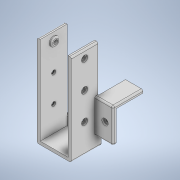
# Autodesk Inventor part: cornerMountTL_PBF
Saved by Autodesk Inventor 2020 (Build 240168000, 168)
## iProperties
Created: 2020-02-06
Part Number: cornerMountTL_PBF
Material: Generic
Document SubType Name: Modeling
Designer: PAB
Density: 1 g/cm^3
Appearance: Default
Author: PAB
Autodesk Inventor part; units mm, degrees
ref_plane "YZ Plane" through (0, 0, 0) normal (1, 0, 0) x (0, 1, 0)
ref_plane "XZ Plane" through (0, 0, 0) normal (0, 1, 0) x (-1, 0, 0)
ref_plane "XY Plane" through (0, 0, 0) normal (0, 0, 1) x (1, 0, 0)
sketch "Sketch1" plane through (0, 0, 0) normal (0, 1, 0) x (-1, 0, 0)
  line L0 (16.2, 12.7) -> (-16.2, 12.7)
  line L1 (-16.2, 12.7) -> (-16.2, -12.7)
  line L2 (-16.2, -12.7) -> (16.2, -12.7)
  line L3 (16.2, -12.7) -> (16.2, 12.7)
  point P0 (0, 0)
  dimension "d0" = 32.4
  dimension "d1" = 25.4
  constraints: 8 end point, 2 parallel, 1 horizontal, 1 perpendicular
  measures "d0" distance of L2.end L1.end
  measures "d1" distance of L1.end L0.end
extrude "Extrusion1" add sketch "Sketch1" along normal blind 3
sketch "Sketch2" plane through (0, 3, 0) normal (0, 1, 0) x (1, 0, 0)
  line L0 (-16.2, 12.7) -> (-16.2, -12.7) projected
  line L1 (16.2, 12.7) -> (-16.2, 12.7) projected
  line L2 (-16.2, -12.7) -> (-13.2, -12.7)
  line L3 (-13.2, -12.7) -> (-13.2, 12.7)
  line L4 (-13.2, 12.7) -> (-16.2, 12.7)
  line L5 (-16.2, 12.7) -> (-16.2, -12.7)
  line L6 (-16.2, -12.7) -> (16.2, -12.7) projected
  line L7 (16.2, 12.7) -> (13.2, 12.7)
  line L8 (13.2, 12.7) -> (13.2, -12.7)
  line L9 (13.2, -12.7) -> (16.2, -12.7)
  line L10 (16.2, -12.7) -> (16.2, 12.7)
  point P0 (0, 0)
  dimension "d4" = 3
  dimension "d5" = 3
  constraints: 16 end point, 4 parallel, 2 horizontal, 2 perpendicular, 2 point on line
  measures "d4" distance of L4.end L3.end
  measures "d5" distance of L9.end L8.end
extrude "Extrusion2" add sketch "Sketch2" along normal blind 83.75 contours L1 L3 L2 L0 | L1 L10 L6 L8
sketch "Sketch3" plane through (16.2, 0, 12.7) normal (1, 0, 0) x (0, 0, -1)
  circle A0 centre (12.7, 79.25) radius 2
  point P0 (12.7, 0)
  dimension "d8" = 4
  constraints: 1 centre point
  measures "d8" diameter of A0
extrude "Extrusion3" cut sketch "Sketch3" against normal blind 3
sketch "Sketch4" plane through (16.2, 0, 12.7) normal (1, 0, 0) x (0, 0, -1)
  circle A0 centre (12.7, 79.25) radius 2 projected
  circle A1 centre (12.7, 79.25) radius 3
  point P0 (12.7, 0)
  dimension "d11" = 6
  constraints: 1 centre point, 1 coincident
  measures "d11" diameter of A1
extrude "Extrusion4" cut sketch "Sketch4" against normal blind 1.5 contours A0 | A1
sketch "Sketch5" plane through (13.2, 3, -12.7) normal (-1, 0, 0) x (0, 0, 1)
  circle A0 centre (12.7, 76.25) radius 2 projected
  circle A1 centre (12.7, 76.25) radius 4.25
  point P0 (12.7, -3)
  dimension "d14" = 8.5
  constraints: 1 centre point, 1 coincident
  measures "d14" diameter of A1
extrude "Extrusion5" add sketch "Sketch5" along normal blind 2
fillet "Fillet1" radius 1.2 1 edges at (11.2, 79.25, -4.25)
pattern_linear "Rectangular Pattern1" count 3 spacing -26 along (0, 1, 0) of "Extrusion3", "Extrusion4"
mirror "Mirror2" about plane through (0, 0, 0) normal (1, 0, 0) of "Extrusion3", "Extrusion4", "Extrusion5", "Fillet1", "Rectangular Pattern1"
sketch "Sketch6" plane through (16.2, 0, 12.7) normal (1, 0, 0) x (0, 0, -1)
  line L0 (25.4, 0) -> (25.4, 86.75) projected
  line L1 (25.4, 43.45) -> (22.4, 43.45)
  line L2 (22.4, 43.45) -> (22.4, 11.05)
  line L3 (22.4, 11.05) -> (25.4, 11.05)
  line L4 (25.4, 11.05) -> (25.4, 43.45)
  point P0 (12.7, 0)
  dimension "d21" = 3
  dimension "d22" = 32.4
  constraints: 8 end point, 2 parallel, 1 horizontal, 1 perpendicular, 1 point on line
  measures "d21" distance of L3.end L2.end
  measures "d22" distance of L2.end L1.end
extrude "Extrusion6" add sketch "Sketch6" along normal blind 17.3
sketch "Sketch7" plane through (16.2, 11.05, -9.7) normal (0, 0, 1) x (1, 0, 0)
  circle A0 centre (9.8, 16.2) radius 2
  point P0 (-16.2, -11.05)
  dimension "d25" = 4
  constraints: 1 centre point
  measures "d25" diameter of A0
extrude "Extrusion7" cut sketch "Sketch7" against normal blind 3
sketch "Sketch8" plane through (16.2, 11.05, -9.7) normal (0, 0, 1) x (1, 0, 0)
  circle A0 centre (9.8, 16.2) radius 2 projected
  circle A1 centre (9.8, 16.2) radius 3
  point P0 (-16.2, -11.05)
  dimension "d28" = 6
  constraints: 1 centre point, 1 coincident
  measures "d28" diameter of A1
extrude "Extrusion8" cut sketch "Sketch8" against normal blind 1.5
sketch "Sketch9" plane through (16.2, 0, -12.7) normal (0, 0, -1) x (-1, 0, 0)
  circle A0 centre (-9.8, 27.25) radius 2 projected
  circle A1 centre (-9.8, 27.25) radius 4.25
  point P0 (16.2, 0)
  dimension "d31" = 8.5
  constraints: 1 centre point, 1 coincident
  measures "d31" diameter of A1
extrude "Extrusion9" add sketch "Sketch9" along normal blind 2
fillet "Fillet2" radius 1.5 1 edges at (30.25, 27.25, -14.7)
sketch "Sketch11" plane through (16.2, 0, -12.7) normal (0, 0, -1) x (-1, 0, 0)
  line L0 (0, 11.05) -> (-17.3, 11.05) projected
  line L1 (0, 11.05) -> (32.4, 11.05)
  line L2 (32.4, 11.05) -> (32.4, 0)
  line L3 (32.4, 0) -> (0, 0)
  line L4 (0, 0) -> (0, 11.05)
  point P0 (16.2, 0)
  constraints: 8 end point, 2 parallel, 1 horizontal, 1 perpendicular
extrude "Extrusion11" add sketch "Sketch11" along normal blind 3
sketch "Sketch14" plane through (33.5, 43.45, -12.7) normal (0, 0, -1) x (-1, 0, 0)
  line L0 (17.3, 0) -> (0, 0) projected
  line L1 (0, 0) -> (16.5, 0)
  line L2 (16.5, 0) -> (16.5, -3)
  line L3 (16.5, -3) -> (0, -3)
  line L4 (0, -3) -> (0, 0)
  point P0 (33.5, -43.45)
  dimension "d48" = 16.5
  dimension "d49" = 3
  constraints: 8 end point, 2 parallel, 1 horizontal, 1 perpendicular
  measures "d48" distance of L2.end L3.end
  measures "d49" distance of L1.end L2.end
extrude "Extrusion14" add sketch "Sketch14" along normal blind 25.4
mirror "Mirror4" about plane through (0, 0, 0) normal (1, 0, 0) of "Extrusion6", "Extrusion7", "Extrusion8", "Extrusion9", "Fillet2", "Extrusion14"
fillet "Fillet5" radius 1.5 15 edges at (33.5, 43.45, -23.9) (33.5, 27.25, -9.7) (24.85, 43.45, -9.7) (24.85, 11.05, -9.7) (-33.5, 43.45, -23.9) (-24.85, 43.45, -9.7) (16.2, 86.75, 0) (-16.2, 86.75, 0) (0, 0, -15.7) (16.2, 0, -1.5) (-33.5, 27.25, -9.7) (-24.85, 11.05, -9.7) (-33.5, 11.05, -11.2) (33.5, 11.05, -11.2) (-16.2, 0, -1.5)
sketch "Sketch15" plane through (-32, 12.55, -9.7) normal (0, 0, 1) x (1, 0, 0)
  line L0 (15.8, 30.9) -> (15.8, 72.7) projected
  line L1 (15.8, 34.925) -> (-11.1125, 34.925)
  line L2 (-11.1125, 34.925) -> (-11.1125, -6.35)
  line L3 (-11.1125, -6.35) -> (15.8, -6.35)
  line L4 (15.8, -6.35) -> (15.8, 34.925)
  point P0 (32, -12.55)
  point P1 (15.8, 49.7)
  point P2 (15.8, 30.9)
  constraints: 8 end point, 2 parallel, 1 horizontal, 1 perpendicular, 1 point on line
extrude "Extrusion15" cut sketch "Sketch15" against normal blind 40
body "Solid1"
